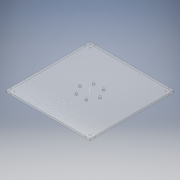
# Autodesk Inventor part: BT403_trajan20_21
Saved by Autodesk Inventor 2022.2 (Build 262287000, 287)
## iProperties
Company: HTBLA Kaindorf
RuleStatus: InUse
Created: 2022-08-21
Part Number: BT403_trajan20_21
Project: Zeichenmaschine_v2
Material: Acryl
Description: papierplatte_plexi
Document SubType Name: Modeling
Designer: trajan20
Density: 1.188 g/cm^3
Appearance: Transparent - farblos
Mass: 260.966 g
Surface Area: 933.292 cm^2
Volume: 219.668 cm^3
AfterDocNew0: iProperties-Editor_aufrufen
Author: jan
Keywords: 2021
Autodesk Inventor part; units mm, degrees
sketch "Skizze3" plane through (0, 0, 0) normal (0, 0, 1) x (1, 0, 0)
  line L0 (0, 0) -> (-210, 0)
  line L1 (-210, 0) -> (-210, 210)
  line L2 (-210, 210) -> (0, 210)
  line L3 (0, 210) -> (0, 0)
  line L4 (0, 0) -> (-210, 210) construction
  line L5 (-210, 0) -> (0, 210) construction
  circle A0 centre (-105, 80) radius 2.5
  line L6 (-105, 58.1482) -> (-105, 151.8518) construction
  point P0 (-105, 105)
  point P1 (-105, 105)
  dimension "d4" = 210
  dimension "d5" = 210
  dimension "d10" = 5
  dimension "d11" = 25
  constraints: 14 end point, 3 midpoint, 2 parallel, 1 centre point, 1 horizontal, 1 perpendicular, 1 point on line, 1 vertical
  measures "d4" distance between parallel lines of L2 L0
  measures "d5" distance between parallel lines of L1 L3
  measures "d10" diameter of A0
  measures "d11" distance of A0.centre point (-105, 105)
extrude "Extrusion3" add sketch "Skizze3" along normal blind 5 contours L0 L1 L2 L3 | A0
fillet "Rundung1" radius 1 4 edges at (-210, 210, 2.5) (-210, 0, 2.5) (0, 0, 2.5) (0, 210, 2.5)
extrude "Extrusion4" cut sketch "Skizze3" along normal blind 4 contours A0
chamfer "Fase1" distance 0.5 angle 45 1 edges at (-107.5, 80, 0)
pattern_circular "Runde Anordnung1" count 6 over 360 about axis through (-105, 105, 0) along (0, 0, 1) of "Extrusion4", "Fase1"
sketch "Skizze5" plane through (-209, 0, 0) normal (0, -1, 0) x (1, 0, 0)
  line L0 (-1, 5) -> (-1, 0) projected
  line L1 (0, 0) -> (208, 0) projected
  line L2 (-2.4185, 2.5) -> (7.6142, 2.5) construction
  point P0 (209, 0)
  point P1 (11, 2.5)
  point P2 (-1, 2.5)
  dimension "d21" = 12
  constraints: 2 end point, 2 point on line, 1 horizontal, 1 midpoint
  measures "d21" distance from line of L0 point (11, 2.5)
ref_plane "Arbeitsebene2" through (-210, 0, 2.5) normal (-0.7054, 0.7088, 0) x (0.7088, 0.7054, 0)
hole "Bohrung1" at (-198, 0, 2.5) direction (0, 1, 0) diameter 2.459 depth 8.8 tip angle 118 thread size "M3x0.5" class "6H" standard "ISO Metric profile"
mirror "Spiegeln2" about plane through (-210, 0, 2.5) normal (-0.7054, 0.7088, 0) of "Bohrung1"
ref_plane "Arbeitsebene3" through (-105, 0, 5) normal (1, 0, 0) x (0, 1, 0)
ref_plane "Arbeitsebene4" through (-210, 105, 5) normal (0, -1, 0) x (1, 0, 0)
mirror "Spiegeln3" about plane through (-105, 0, 5) normal (1, 0, 0) of "Bohrung1", "Spiegeln2"
mirror "Spiegeln4" about plane through (-210, 105, 5) normal (0, -1, 0) of "Bohrung1", "Spiegeln2", "Spiegeln3"
equation "\"d5\" = d4"
